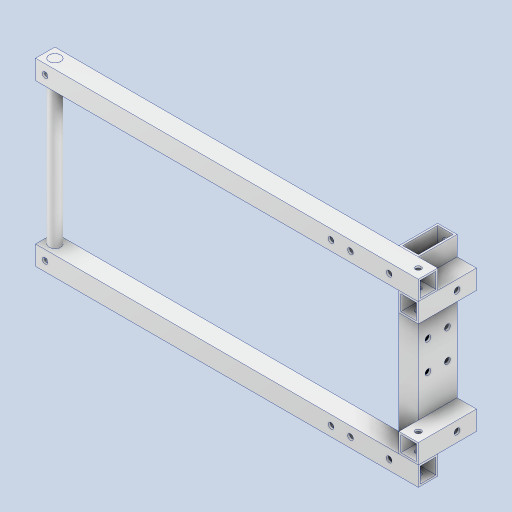
# Autodesk Inventor part: ballhand-v2-ASP-H
Saved by Autodesk Inventor 2024 (Build 280153000, 153)
## iProperties
Created: 2024-03-16
Part Number: ballhand-v2-ASP-H
Material: アルミニウム 6061
Document SubType Name: Modeling
Designer: haruy
Density: 2.7 g/cm^3
Appearance: アルミニウム - フラット
Author: haruy
Autodesk Inventor part; units mm, degrees
ref_plane "YZ Plane" through (0, 0, 0) normal (1, 0, 0) x (0, 1, 0)
ref_plane "XZ Plane" through (0, 0, 0) normal (0, 1, 0) x (-1, 0, 0)
ref_plane "XY Plane" through (0, 0, 0) normal (0, 0, 1) x (1, 0, 0)
derived "ballhand-v2-Sketch-Base.ipt"
sketch "横から" plane through (0, 0, 0) normal (0, 0, 1) x (1, 0, 0)
  circle A0 centre (0, 0) radius 95
  line L0 (-321.6558, -95) -> (545.18, -95)
  line L1 (95, 81) -> (293, 81)
  line L2 (293, 81) -> (293, 61)
  line L3 (293, 61) -> (95, 61)
  line L4 (95, 61) -> (95, 81)
  line L5 (-52.5, 46.5) -> (145, 46.5)
  line L6 (145, 46.5) -> (145, 36.5)
  line L7 (145, 36.5) -> (-52.5, 36.5)
  line L8 (-52.5, 36.5) -> (-52.5, 46.5)
  line L9 (-52.5, -36.5) -> (145, -36.5)
  line L10 (145, -36.5) -> (145, -46.5)
  line L11 (145, -46.5) -> (-52.5, -46.5)
  line L12 (-52.5, -46.5) -> (-52.5, -36.5)
  line L13 (-50.5, 46.5) -> (-44.5, 46.5)
  line L14 (-44.5, 46.5) -> (-44.5, -46.5)
  line L15 (-44.5, -46.5) -> (-50.5, -46.5)
  line L16 (-50.5, -46.5) -> (-50.5, 46.5)
  line L17 (95, 5) -> (115, 5)
  line L18 (115, 5) -> (115, -5)
  line L19 (115, -5) -> (95, -5)
  line L20 (95, -5) -> (95, 5)
  line L21 (115, 4.5) -> (117.2, 4.5)
  line L22 (117.2, 4.5) -> (117.2, -4.5)
  line L23 (117.2, -4.5) -> (115, -4.5)
  line L24 (115, -4.5) -> (115, 4.5)
  line L25 (117.2, 10) -> (125, 10)
  line L26 (125, 10) -> (125, -10)
  line L27 (125, -10) -> (117.2, -10)
  line L28 (117.2, -10) -> (117.2, 10)
  line L29 (125, 46.5) -> (135, 46.5)
  line L30 (135, 46.5) -> (135, -46.5)
  line L31 (135, -46.5) -> (125, -46.5)
  line L32 (125, -46.5) -> (125, 46.5)
  line L33 (135, 36.5) -> (145, 36.5)
  line L34 (145, 36.5) -> (145, 26.5)
  line L35 (145, 26.5) -> (135, 26.5)
  line L36 (135, 26.5) -> (135, 36.5)
  line L37 (135, -36.5) -> (145, -36.5)
  line L38 (145, -36.5) -> (145, -26.5)
  line L39 (145, -26.5) -> (135, -26.5)
  line L40 (135, -26.5) -> (135, -36.5)
  line L41 (95, 33) -> (115, 33)
  line L42 (115, 33) -> (115, 43)
  line L43 (115, 43) -> (95, 43)
  line L44 (95, 43) -> (95, 33)
  line L45 (0, 0) -> (115, 0)
  line L46 (95, -33) -> (115, -33)
  line L47 (115, -43) -> (95, -43)
  line L48 (95, -43) -> (95, -33)
  line L49 (115, -33) -> (115, -43)
  line L50 (115, 81) -> (125, 81)
  line L51 (125, 81) -> (125, -43)
  line L52 (125, -43) -> (115, -43)
  line L53 (115, -43) -> (115, 81)
  circle A1 centre (105, 19) radius 2.5
  point P0 (-47.5, 41.5)
  point P1 (-47.5, -41.5)
  point P2 (130, 41.5)
  point P3 (100, 41.5)
  point P4 (110, 41.5)
  point P5 (130, -41.5)
  point P6 (100, -41.5)
  point P7 (110, -41.5)
  dimension "d1" = 5
  dimension "d2" = 5
  dimension "d3" = 5
  dimension "d4" = 5
  dimension "d5" = 5
  dimension "d6" = 5
  dimension "d7" = 5
  dimension "d8" = 5
  dimension "d9" = 5
  dimension "d10" = 5
  measures "d1" distance from line of point (-47.5, 41.5) L5
  measures "d2" distance from line of L8 point (-47.5, 41.5)
  measures "d3" distance from line of L9 point (-47.5, -41.5)
  measures "d4" distance from line of L12 point (-47.5, -41.5)
  measures "d5" distance from line of point (130, 41.5) L30
  measures "d6" distance from line of point (130, 41.5) L5
  measures "d7" horizontal distance of point (100, 41.5) A1.centre
  measures "d8" horizontal distance of A1.centre point (110, 41.5)
  measures "d9" distance from line of point (100, 41.5) L5
  measures "d10" distance from line of point (110, 41.5) L5
extrude "押し出し1" add sketch "横から" along normal blind 10 contours L7 L14 L5 A0 | A0 L5 L53 L43 L44 L7 | L44 L43 L42 L7 | L7 L16 L5 L14 | L5 L32 L7 L42 L53 | L7 L8 L5 L16 | L5 L30 L7 L32 | L5 L6 L7 L30
extrude "押し出し2" add sketch "横から" along normal blind 10 separate body contours L9 L48 L47 L52 L32 L11 A0 | A0 L11 L14 L9 | L14 L11 L16 L9 | L9 L49 L47 L48 | L32 L9 L30 L11 | L16 L11 L12 L9 | L9 L32 L52 L49 | L30 L9 L10 L11
extrude "押し出し3" add sketch "横から" along normal blind 10 and the other way blind 20 separate body contours L7 L34 L35 L30
extrude "押し出し4" add sketch "横から" along normal blind 10 and the other way blind 20 separate body contours L30 L39 L38 L9
extrude "押し出し5" add sketch "横から" against normal blind 20 separate body contours L32 L9 L30 L11 | L5 L30 L7 L32 | L7 L30 L9 L32 L26
shell "シェル1" thickness 1 removed faces 10 at (145, 39.8333, 3.3333) at (141.6667, 29.8333, 10) at (141.6667, 29.8333, -20) at (131.6667, 46.5, -6.6667) at (128.3333, -46.5, -6.6667) at (138.3333, -33.1667, -20) at (138.3333, -33.1667, 10) at (145, -43.1667, 3.3333) at (-52.5, -39.8333, 3.3333) at (-52.5, 43.1667, 3.3333) bodies 1 3 5 4 2
hole "穴1" at (-47.5, -41.5, 0) at (130, 41.5, 0) at (100, 41.5, 0) at (110, 41.5, 0) at (100, -41.5, 0) at (110, -41.5, 0) at (130, -41.5, 0) at (-47.5, 41.5, 0) direction (0, 0, 1) diameter 3 end through all both bodies 1 2 5
sketch "スケッチ2" plane through (-52.5, -46.5, 0) normal (0, -1, 0) x (1, 0, 0)
  line L0 (0, 10) -> (197.5, 10) projected
  line L1 (0, 0) -> (0, 10) projected
  line L2 (197.5, 0) -> (197.5, 10) projected
  circle A0 centre (5, 5) radius 3
  point P0 (52.5, 0)
  point P1 (192.5, 5)
  dimension "d33" = 5
  dimension "d34" = 5
  dimension "d35" = 5
  dimension "d36" = 5
  dimension "d51" = 6
  constraints: 1 centre point, 1 coincident
  measures "d33" distance from line of point (5, 5) L0
  measures "d34" distance from line of L1 point (5, 5)
  measures "d35" distance from line of point (192.5, 5) L0
  measures "d36" distance from line of L2 point (192.5, 5)
  measures "d51" diameter of A0
hole "穴2" at (140, -46.5, 5) direction (0, 1, 0) diameter 3 end through all both bodies 2 4 3 1
hole "穴3" at (-47.5, -46.5, 5) direction (0, 1, 0) diameter 6 end through all both bodies 2 1
extrude "押し出し6" add sketch "スケッチ2" against normal up to surface (93 mm away) separate body
sketch "スケッチ3" plane through (125, -46.5, 0) normal (-1, 0, 0) x (0, 0, 1)
  line L0 (-20, 0) -> (-20, 93) projected
  line L1 (-20, 20) -> (10, 20) projected
  line L2 (-20, 83) -> (10, 83) projected
  line L3 (-20, 46.5) -> (0, 46.5)
  point P0 (-10, 78)
  point P1 (-10, 15)
  point P2 (-15, 54)
  point P3 (-5, 54)
  point P4 (-15, 39)
  point P5 (-5, 39)
  dimension "d54" = 10
  dimension "d55" = 5
  dimension "d56" = 10
  dimension "d57" = 5
  dimension "d58" = 10
  dimension "d59" = 7.5
  dimension "d60" = 7.5
  dimension "d61" = 5
  constraints: 2 end point, 2 symmetric about line, 1 horizontal, 1 midpoint
  measures "d54" distance from line of point (-10, 15) L0
  measures "d55" distance from line of point (-10, 15) L1
  measures "d56" distance from line of L0 point (-10, 78)
  measures "d57" distance from line of point (-10, 78) L2
  measures "d58" distance of point (-5, 54) point (-15, 54)
  measures "d59" distance from line of point (-15, 54) L3
  measures "d60" distance from line of point (-5, 54) L3
  measures "d61" distance from line of point (-15, 54) L0
hole "穴4" at (125, 31.5, -10) at (125, -31.5, -10) at (125, 7.5, -15) at (125, 7.5, -5) at (125, -7.5, -15) at (125, -7.5, -5) direction (1, 0, 0) diameter 3 end through all bodies 5 3 4
equation "\"d8\" = d7"
equation "\"d9\" = d7"
equation "\"d10\" = d7"
equation "\"d60\" = d59"
